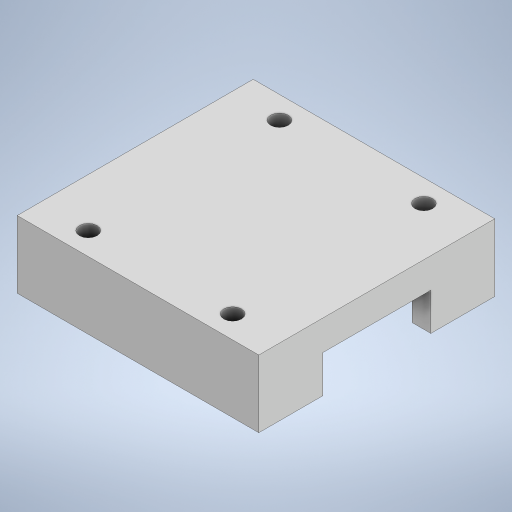
# Autodesk Inventor part: Part1
Saved by Autodesk Inventor 2024 (Build 280153000, 153)
## iProperties
Created: 2023-07-25
Part Number: Part1
Material: Generic
Document SubType Name: Modeling
Designer: 18179
Density: 1 g/cm^3
Appearance: Default
Author: 18179
Autodesk Inventor part; units mm, degrees
ref_plane "YZ Plane" through (0, 0, 0) normal (1, 0, 0) x (0, 1, 0)
ref_plane "XZ Plane" through (0, 0, 0) normal (0, 1, 0) x (-1, 0, 0)
ref_plane "XY Plane" through (0, 0, 0) normal (0, 0, 1) x (1, 0, 0)
derived "ESC_Mount.ipt"
sketch "Sketch12" plane through (0, 2.54, 0) normal (0, 1, 0) x (1, 0, 0)
  line L0 (1.3335, -3.8735) -> (-33.3375, -3.8735) projected
  line L1 (-33.3375, -0.635) -> (-33.3375, -3.8735) projected
  line L2 (-33.3375, -0.635) -> (1.3335, -0.635) projected
  line L3 (1.3335, -3.8735) -> (1.3335, -0.635) projected
  line L4 (-36.5125, -11.4935) -> (4.5085, -11.4935) projected
  line L5 (4.5085, -11.4935) -> (4.5085, 28.575) projected
  line L6 (4.5085, 28.575) -> (-36.5125, 28.575) projected
  line L7 (-36.5125, 28.575) -> (-36.5125, -11.4935) projected
  circle A0 centre (-3.7465, -7.6835) radius 1.5 projected
  circle A1 centre (-28.2575, -7.6835) radius 1.5 projected
  line L8 (1.3335, 17.7165) -> (1.3335, 20.955) projected
  line L9 (1.3335, 17.7165) -> (-33.3375, 17.7165) projected
  line L10 (-33.3375, 20.955) -> (-33.3375, 17.7165) projected
  line L11 (-33.3375, 20.955) -> (1.3335, 20.955) projected
  circle A2 centre (-28.2575, 24.7777) radius 1.5 projected
  circle A3 centre (-3.7465, 24.7777) radius 1.5 projected
  line L12 (-26.9875, 16.383) -> (-26.9875, 19.685) projected
  line L13 (-26.9875, 16.383) -> (-5.0165, 16.383) projected
  line L14 (-5.0165, 19.685) -> (-5.0165, 16.383) projected
  line L15 (-26.9875, 19.685) -> (-5.0165, 19.685) projected
  line L16 (-5.0165, -2.6035) -> (-26.9875, -2.6035) projected
  line L17 (-5.0165, 0.6985) -> (-5.0165, -2.6035) projected
  line L18 (-5.0165, 0.6985) -> (-26.9875, 0.6985) projected
  line L19 (-26.9875, -2.6035) -> (-26.9875, 0.6985) projected
  point P0 (0, 0)
  point P1 (-26.9875, -0.635)
  point P2 (-5.0165, -0.635)
  point P3 (-5.0165, 17.7165)
  point P4 (-26.9875, 17.7165)
extrude "Extrusion1" add sketch "Sketch12" along normal blind 6.35
sketch "Sketch2" plane through (-36.5125, 8.89, -28.575) normal (0, 1, 0) x (1, 0, 0)
  circle A0 centre (8.255, -36.2585) radius 1.5 projected
  circle A1 centre (8.255, -36.2585) radius 3.175
  circle A2 centre (8.255, -3.7973) radius 1.5 projected
  circle A3 centre (8.255, -3.7973) radius 3.175
  circle A4 centre (32.766, -3.7973) radius 1.5 projected
  circle A5 centre (32.766, -3.7973) radius 3.175
  circle A6 centre (32.766, -36.2585) radius 1.5 projected
  circle A7 centre (32.766, -36.2585) radius 3.175
  line L0 (41.021, -40.0685) -> (41.021, 0) projected
  line L1 (41.021, 0) -> (0, 0) projected
  line L2 (0, 0) -> (0, -40.0685) projected
  line L3 (0, -40.0685) -> (41.021, -40.0685) projected
  circle A8 centre (32.766, -36.2585) radius 1.5 projected
  circle A9 centre (8.255, -36.2585) radius 1.5 projected
  circle A10 centre (8.255, -3.7973) radius 1.5 projected
  circle A11 centre (32.766, -3.7973) radius 1.5 projected
  line L4 (37.846, -29.21) -> (37.846, -32.4485) projected
  line L5 (37.846, -32.4485) -> (3.175, -32.4485) projected
  line L6 (3.175, -32.4485) -> (3.175, -29.21) projected
  line L7 (3.175, -29.21) -> (9.525, -29.21) projected
  line L8 (9.525, -29.21) -> (9.525, -27.8765) projected
  line L9 (9.525, -27.8765) -> (31.496, -27.8765) projected
  line L10 (31.496, -27.8765) -> (31.496, -29.21) projected
  line L11 (31.496, -29.21) -> (37.846, -29.21) projected
  line L12 (37.846, -7.62) -> (37.846, -10.8585) projected
  line L13 (37.846, -10.8585) -> (31.496, -10.8585) projected
  line L14 (31.496, -10.8585) -> (31.496, -12.192) projected
  line L15 (31.496, -12.192) -> (9.525, -12.192) projected
  line L16 (9.525, -12.192) -> (9.525, -10.8585) projected
  line L17 (9.525, -10.8585) -> (3.175, -10.8585) projected
  line L18 (3.175, -10.8585) -> (3.175, -7.62) projected
  line L19 (3.175, -7.62) -> (37.846, -7.62) projected
  line L20 (3.175, -36.8935) -> (3.175, -3.175)
  line L21 (3.175, -3.175) -> (37.846, -3.175)
  line L22 (37.846, -3.175) -> (37.846, -36.8935)
  line L23 (37.846, -36.8935) -> (3.175, -36.8935)
  line L24 (3.175, -10.8585) -> (0, -10.8585)
  line L25 (9.525, -10.8585) -> (3.175, -10.8585) projected
  line L26 (3.175, -29.21) -> (0, -29.21)
  line L27 (37.846, -29.21) -> (41.021, -29.21)
  line L28 (37.846, -10.8585) -> (41.021, -10.8585)
  point P0 (36.5125, -28.575)
  point P1 (5.1416, -3.175)
  point P2 (5.1441, -36.8935)
  point P3 (11.3659, -36.8935)
  point P4 (29.6551, -36.8935)
  point P5 (35.8769, -36.8935)
  point P6 (35.8794, -3.175)
  point P7 (29.6526, -3.175)
  point P8 (11.3684, -3.175)
  dimension "d3" = 6.35
  dimension "d4" = 6.35
  dimension "d5" = 6.35
  dimension "d6" = 6.35
  dimension "d7" = 3.175
  constraints: 16 end point, 6 point on line, 4 centre point, 4 coincident, 1 collinear, 1 perpendicular, 3 other
  measures "d3" diameter of A1
  measures "d4" diameter of A3
  measures "d5" diameter of A5
  measures "d6" diameter of A7
  measures "d7" distance between parallel lines of L2 L20
extrude "Extrusion2" cut sketch "Sketch2" against normal through all contours A0 L23 | A0 L23 A1 | L23 A0 | A0 L23 A1 | L23 L20 L5 L22 A7 A1 | L23 A6 A7 | A7 L23 A6 | L6 L7 L8 L9 L10 L11 L4 L5 | L23 A6 | A6 L23 | L20 L17 L16 L15 L14 L13 L22 L11 L10 L9 L8 L7 | L26 L2 L24 L20 | L22 L28 L0 L27 | L18 L19 L12 L13 L14 L15 L16 L17 | L20 L21 A3 A5 L22 L19 | L21 A2 A3 | A3 L21 A2 | L21 A4 A5 | A5 L21 A4 | L21 A2 | A2 L21 | L21 A4 | A4 L21
sketch "Sketch3" plane through (-36.5125, 8.89, 11.4935) normal (0, 1, 0) x (1, 0, 0)
  line L0 (37.846, 29.21) -> (41.021, 29.21) projected
  line L1 (41.021, 29.21) -> (41.021, 40.0685) projected
  line L2 (41.021, 40.0685) -> (0, 40.0685) projected
  line L3 (0, 40.0685) -> (0, 29.21) projected
  line L4 (0, 29.21) -> (3.175, 29.21) projected
  line L5 (3.175, 29.21) -> (3.175, 36.8935) projected
  line L6 (3.175, 36.8935) -> (5.1416, 36.8935) projected
  arc A0 (11.3684, 36.8935) -> (5.1416, 36.8935) centre (8.255, 36.2712) ccw projected
  line L7 (11.3684, 36.8935) -> (29.6526, 36.8935) projected
  arc A1 (35.8794, 36.8935) -> (29.6526, 36.8935) centre (32.766, 36.2712) ccw projected
  line L8 (35.8794, 36.8935) -> (37.846, 36.8935) projected
  line L9 (37.846, 36.8935) -> (37.846, 29.21) projected
  line L10 (37.846, 10.8585) -> (37.846, 3.175) projected
  line L11 (37.846, 3.175) -> (35.8769, 3.175) projected
  arc A2 (29.6551, 3.175) -> (35.8769, 3.175) centre (32.766, 3.81) ccw projected
  line L12 (29.6551, 3.175) -> (11.3659, 3.175) projected
  arc A3 (5.1441, 3.175) -> (11.3659, 3.175) centre (8.255, 3.81) ccw projected
  line L13 (5.1441, 3.175) -> (3.175, 3.175) projected
  line L14 (3.175, 3.175) -> (3.175, 10.8585) projected
  line L15 (3.175, 10.8585) -> (0, 10.8585) projected
  line L16 (0, 10.8585) -> (0, 0) projected
  line L17 (0, 0) -> (41.021, 0) projected
  line L18 (41.021, 0) -> (41.021, 10.8585) projected
  line L19 (41.021, 10.8585) -> (37.846, 10.8585) projected
  line L20 (0, 29.21) -> (3.175, 29.21)
  line L21 (3.175, 29.21) -> (3.175, 10.8585)
  line L22 (3.175, 10.8585) -> (0, 10.8585)
  line L23 (0, 10.8585) -> (0, 29.21)
  line L24 (37.846, 29.21) -> (41.021, 29.21)
  line L25 (41.021, 29.21) -> (41.021, 10.8585)
  line L26 (41.021, 10.8585) -> (37.846, 10.8585)
  line L27 (37.846, 10.8585) -> (37.846, 29.21)
  point P0 (36.5125, 11.4935)
  constraints: 16 end point, 6 equal length, 2 perpendicular
extrude "Extrusion3" add sketch "Sketch3" along normal blind 2.54 contours L9 L8 A1 L7 A0 L6 L5 L4 L3 L2 L1 L0 | L0 L25 L19 L27 | L19 L18 L17 L16 L15 L14 L13 A3 L12 A2 L11 L10 | L4 L21 L15 L23
sketch "Sketch4" plane through (-36.5125, 11.43, 11.4935) normal (0, 1, 0) x (1, 0, 0)
  line L0 (0, 40.0685) -> (0, 0) projected
  line L1 (0, 0) -> (41.021, 0) projected
  line L2 (41.021, 0) -> (41.021, 40.0685) projected
  line L3 (41.021, 40.0685) -> (0, 40.0685) projected
  line L4 (3.175, 3.175) -> (3.175, 36.8935) projected
  line L5 (3.175, 36.8935) -> (5.1416, 36.8935) projected
  arc A0 (11.3684, 36.8935) -> (5.1416, 36.8935) centre (8.255, 36.2712) ccw projected
  line L6 (11.3684, 36.8935) -> (29.6526, 36.8935) projected
  arc A1 (35.8794, 36.8935) -> (29.6526, 36.8935) centre (32.766, 36.2712) ccw projected
  line L7 (35.8794, 36.8935) -> (37.846, 36.8935) projected
  line L8 (37.846, 36.8935) -> (37.846, 3.175) projected
  line L9 (37.846, 3.175) -> (35.8769, 3.175) projected
  arc A2 (29.6551, 3.175) -> (35.8769, 3.175) centre (32.766, 3.81) ccw projected
  line L10 (29.6551, 3.175) -> (11.3659, 3.175) projected
  arc A3 (5.1441, 3.175) -> (11.3659, 3.175) centre (8.255, 3.81) ccw projected
  line L11 (5.1441, 3.175) -> (3.175, 3.175) projected
  circle A4 centre (8.255, 36.2712) radius 1.5
  circle A5 centre (32.766, 36.2712) radius 1.5
  circle A6 centre (32.766, 3.81) radius 1.5
  circle A7 centre (8.255, 3.81) radius 1.5
  point P0 (36.5125, 11.4935)
  dimension "d12" = 3
  dimension "d13" = 3
  dimension "d14" = 3
  dimension "d15" = 3
  constraints: 4 centre point, 4 coincident
  measures "d12" diameter of A4
  measures "d13" diameter of A5
  measures "d14" diameter of A6
  measures "d15" diameter of A7
extrude "Extrusion4" add sketch "Sketch4" along normal blind 2.54 contours L3 L2 L1 L0 | L4 L5 A0 L6 A1 L7 L8 L9 A2 L10 A3 L11
body "Solid1"
